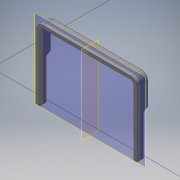
# Autodesk Inventor part: atmega_pin
Saved by Autodesk Inventor 2018 (Build 220112000, 112)
## iProperties
Created: 2017-04-13
Part Number: atmega_pin
Material: Generic
Document SubType Name: Sheet Metal
Designer: kampe_000
Density: 1 g/cm^3
Sheet Metal Rule: Default_mm
Appearance: Default
Author: kampe_000
Autodesk Inventor part; units mm, degrees
ref_plane "YZ Plane" through (0, 0, 0) normal (1, 0, 0) x (0, 1, 0)
ref_plane "XZ Plane" through (0, 0, 0) normal (0, 1, 0) x (-1, 0, 0)
ref_plane "XY Plane" through (0, 0, 0) normal (0, 0, 1) x (1, 0, 0)
sketch "Sketch1" plane through (0, 0, 0) normal (0, 1, 0) x (-1, 0, 0)
  line L0 (-4.5709, 0.1557) -> (-12.5709, 0.1557)
  line L1 (-12.5709, 0.1557) -> (-12.5709, 1.3557)
  line L2 (-12.5709, 1.3557) -> (-4.5709, 1.3557)
  line L3 (-4.5709, 1.3557) -> (-4.5709, 0.1557)
  dimension "d27" = 8
  dimension "d28" = 1.2
  measures "d27" distance of L1.end L2.end
  measures "d28" distance of L0.end L1.end
extrude "Plate4" add sketch "Sketch1" along normal blind 0.25
sketch "Sketch5" plane through (12.3209, 0.25, 1.3557) normal (1, 0, 0) x (0, 1, 0)
  line L0 (0, -1.2) -> (0, 0)
  line L1 (0, 0) -> (-5.7, 0)
  line L2 (-5.7, 0) -> (-5.7, -1.2)
  line L3 (-5.7, -1.2) -> (0, -1.2)
  constraints: 6 end point, 1 horizontal, 1 perpendicular, 1 vertical
edge flange "Flange4" height 5.7 angle 90 thickness 0.25 bend radius 0.25 thickness toward (1, 0, 0) relief tear relief width 0.25 relief depth 0.125 corner gap 0.25 corner form 0 edges at (12.5709, 0, 0.7557) (4.5709, 0, 0.7557) wall of the first edge with corners at (12.3209, 0.25, 0.1557) (12.3209, 0.25, 1.3557) (12.3209, -5.45, 1.3557) (12.3209, -5.45, 0.1557)
bend "Bend4"
corner "Corner4"
sketch "Sketch6" plane through (12.5709, -5.45, 1.3557) normal (1, 0, 0) x (0, 0, -1)
  line L0 (1.2, 0) -> (0, 0) projected
  line L1 (0.6, 0) -> (0.6, 5.2) construction
  line L2 (1.2, 5.2) -> (0, 5.2) projected
  line L3 (1.2, 3.4021) -> (0.85, 3.2)
  line L4 (0.85, 3.2) -> (0.85, 0)
  line L5 (1.2, 0) -> (0.85, 0)
  line L6 (1.2, 5.2) -> (1.2, 0) projected
  line L7 (1.2, 3.4021) -> (1.2, 0)
  line L8 (0, 5.7) -> (1.2, 5.7) projected
  point P0 (1.3557, 5.45)
  dimension "d52" = 3.2
  dimension "d54" = 0.25
  dimension "d56" = 2.5
  constraints: 10 end point, 2 midpoint, 2 point on line, 1 collinear, 1 perpendicular, 1 vertical
  measures "d52" distance of L3.end L4.end
  measures "d54" distance between parallel lines of L1 L4
  measures "d56" distance from line of L3.end L8
extrude "Cut1" cut sketch "Sketch6" against normal blind 0.25
ref_plane "Work Plane1" through (12.5709, -0.25, 0.7557) normal (0, 0, -1) x (-1, 0, 0)
ref_plane "Work Plane2" through (8.5709, -5.45, 1.3557) normal (1, 0, 0) x (0, 0, -1)
mirror "Mirror2" about plane through (8.5709, -5.45, 1.3557) normal (1, 0, 0) of "Cut1"
sketch "Sketch7" plane through (8.5709, -5.45, 1.3557) normal (1, 0, 0) x (0, 0, -1)
  line L0 (0, 0) -> (0.85, 0) projected
  line L1 (0, 5.7) -> (1.2, 5.7) projected
  line L2 (0, 0) -> (0.35, 0)
  line L3 (0.35, 0) -> (0.35, 5.7)
  line L4 (0.35, 5.7) -> (0, 5.7)
  line L5 (0, 5.7) -> (0, 0)
  line L6 (1.2, 5.7) -> (1.2, 5.45) projected
  line L7 (1.2, 5.45) -> (0, 5.45) projected
  line L8 (0, 5.45) -> (0, 5.7) projected
  line L9 (0, 5.7) -> (1.2, 5.7) projected
  line L10 (0.6, 6.84) -> (0.6, -1.14) projected
  point P0 (1.3557, 5.45)
  dimension "d57" = 0.25
  constraints: 8 end point, 2 parallel, 1 horizontal, 1 perpendicular, 1 point on line
  measures "d57" distance between parallel lines of L10 L3
extrude "Cut2" cut sketch "Sketch7" along normal through all both and the other way through all contours L5 L7 L3 L0 | L5 L1 L3 L7
equation "\"d27\" = atmegaPinBaseWidth"
equation "\"d28\" = atmegaPinWidth1"
equation "\"d52\" = atmegaSeatingPlaneDistance"
equation "\"d54\" = 0.5 * atmegaPinWidth2"
equation "\"d50\" = Thickness"
equation "\"d57\" = 0.5 * atmegaPinWidth2"
equation "\"d58\" = Thickness"
equation "\"d29\" = Thickness"
equation "\"d40\" = BendReliefWidth"
equation "\"d41\" = BendReliefDepth"
equation "\"d42\" = MinimumRemnant"
equation "\"d43\" = TransitionRadius"
equation "\"d44\" = atmegaPinLenght"
equation "\"d46\" = BendRadius"
equation "\"d47\" = CornerReliefSize"
equation "\"d48\" = GapSize"
equation "\"d49\" = JacobiRadiusSize"
equation "\"BendRadius\" = Thickness"
equation "\"BendReliefWidth\" = Thickness"
equation "\"BendReliefDepth\" = 0.5 * Thickness"
equation "\"CornerReliefSize\" = 4 * Thickness"
equation "\"MinimumRemnant\" = 2 * Thickness"
equation "\"TransitionRadius\" = BendRadius"
equation "\"JacobiRadiusSize\" = BendRadius"
equation "\"GapSize\" = Thickness"
equation "\"atmegaPinThickness\" = 0.3"
equation "\"atmegaPinWidth1\" = 1.2"
equation "\"atmegaPinWidth2\" = 0.5"
equation "\"atmegaEndPinWidth\" = 0.9"
equation "\"atmegaPinBendAngle\" = 80deg"
equation "\"atmegaPinBaseWidth\" = 8"
equation "\"atmegaSeatingPlaneDistance\" = 3.2"
equation "\"Thickness\" = 0.25"
equation "\"atmegaPinLenght\" = 5.7"
body "Solid2"
